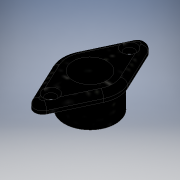
# Autodesk Inventor part: Deck_Bushing_Outer
Saved by Autodesk Inventor 2016 (Build 200138000, 138)
## iProperties
Created: 2016-05-07
Part Number: Deck_Bushing_Outer
Material: Nylon 6/6
Document SubType Name: Modeling
Designer: agmle
Density: 1.13 g/cm^3
Appearance: Rough - Black
Mass: 2.99259 g
Surface Area: 21.2851 cm^2
Volume: 2.64831 cm^3
Cutout_Diameter: 0.748 in
Mount_Hole_Diameter: 0.150 in
Mount_Hole_Spacing: 1.150 in
Author: agmle
Autodesk Inventor part; units mm, degrees
ref_plane "YZ Plane" through (0, 0, 0) normal (1, 0, 0) x (0, 1, 0)
ref_plane "XZ Plane" through (0, 0, 0) normal (0, 1, 0) x (-1, 0, 0)
ref_plane "XY Plane" through (0, 0, 0) normal (0, 0, 1) x (1, 0, 0)
sketch "Sketch1" plane through (0, 0, 0) normal (0, 1, 0) x (-1, 0, 0)
  circle A0 centre (0, 0) radius 9.5
  dimension "Cutout_Diameter" = 19
  constraints: 1 centre point, 1 coincident
  measures "Cutout_Diameter" diameter of A0
extrude "Extrusion1" add sketch "Sketch1" along normal blind 9.2
sketch "Sketch2" plane through (0, 9.2, 0) normal (0, 1, 0) x (1, 0, 0)
  line L0 (0, 0) -> (0, 17.625) construction
  line L1 (0, 0) -> (0, -17.625) construction
  arc A0 (-2.7148, -18.9016) -> (2.7148, -18.9016) centre (0, -17.625) ccw
  arc A1 (2.7148, 18.9016) -> (-2.7148, 18.9016) centre (0, 17.625) ccw
  line L2 (-2.7148, -18.9016) -> (-9.5019, -4.4681)
  line L3 (-9.5019, 4.4681) -> (-2.7148, 18.9016)
  line L4 (2.7148, 18.9016) -> (9.5019, 4.4681)
  line L5 (9.5019, -4.4681) -> (2.7148, -18.9016)
  arc A2 (9.5019, -4.4681) -> (9.5019, 4.4681) centre (0, 0) ccw
  arc A3 (-9.5019, 4.4681) -> (-9.5019, -4.4681) centre (0, 0) ccw
  dimension "Mount_Tip_Radius" = 6
  dimension "Mount_Center_Radius" = 10.5
  dimension "Mount_Tip_Length" = 41.25
  constraints: 14 end point, 8 point on circle, 5 tangent, 4 centre point, 3 coincident, 2 parallel, 2 vertical, 1 collinear, 1 equal radius
  measures "Mount_Tip_Radius" diameter of A1
  measures "Mount_Center_Radius" radius of A3
extrude "Extrusion2" add sketch "Sketch2" along normal blind 3.2
sketch "Sketch3" plane through (0, 12.4, 0) normal (0, 1, 0) x (1, 0, 0)
  line L0 (0, -14.605) -> (0, 14.605) construction
  point P0 (0, 0)
  point P1 (0, 0)
  dimension "Mount_Hole_Spacing" = 29.21
  constraints: 3 coincident, 2 end point, 1 midpoint, 1 vertical
  measures "Mount_Hole_Spacing" distance of L0.start L0.end
hole "Hole1" at (0, 12.4, 14.605) at (0, 12.4, -14.605) direction (0, -1, 0) diameter 3.81 end through all countersink diameter 5.715 countersink angle 82
sketch "Sketch4" plane through (0, 12.4, 0) normal (0, 1, 0) x (1, 0, 0)
  point P0 (0, 0)
  point P1 (0, 0)
  constraints: 1 coincident
hole "Hole2" at (0, 12.4, 0) direction (0, -1, 0) diameter 12.6 end through all
fillet "Fillet1" radius 2 8 edges at (10.5, 12.4, 0) (6.1084, 12.4, -11.6848) (0, 12.4, -20.625) (-6.1084, 12.4, -11.6848) (-10.5, 12.4, 0) (-6.1084, 12.4, 11.6848) (0, 12.4, 20.625) (6.1084, 12.4, 11.6848)
body "Solid1"
